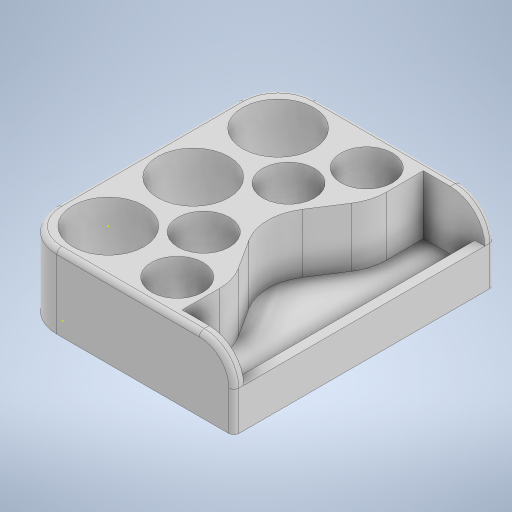
# Autodesk Inventor part: multi_battery_holder
Saved by Autodesk Inventor 2024 (Build 280153000, 153)
## iProperties
Created: 2024-03-18
Part Number: multi_battery_holder
Material: Generic
Document SubType Name: Modeling
Designer: kubad
Density: 1 g/cm^3
Appearance: Default
Author: kubad
Autodesk Inventor part; units mm, degrees
ref_plane "YZ Plane" through (0, 0, 0) normal (1, 0, 0) x (0, 1, 0)
ref_plane "XZ Plane" through (0, 0, 0) normal (0, 1, 0) x (-1, 0, 0)
ref_plane "XY Plane" through (0, 0, 0) normal (0, 0, 1) x (1, 0, 0)
sketch "Sketch1" plane through (0, 0, 0) normal (0, 1, 0) x (-1, 0, 0)
  circle A0 centre (0, 0) radius 7.25
  line L0 (0, -7.25) -> (0, -17.25)
  circle A1 centre (0, -17.25) radius 7.25
  line L1 (0, -24.5) -> (0, -34.5)
  circle A2 centre (0, -34.5) radius 7.25
  line L2 (0, -7.25) -> (0, -10)
  line L3 (0, -24.5) -> (0, -27.25)
  line L4 (0, 7.25) -> (-16, 7.25)
  line L5 (-16, 7.25) -> (-16, 2)
  circle A3 centre (-16, 2) radius 5.25
  line L6 (0, -41.75) -> (-16, -41.75)
  line L7 (-16, -41.75) -> (-16, -36.5)
  circle A4 centre (-16, -36.5) radius 5.25
  line L8 (0, -8.625) -> (-16, -8.625)
  line L9 (0, -25.875) -> (-16, -25.875)
  circle A5 centre (-10.75, -8.625) radius 5.25
  circle A6 centre (-10.75, -25.875) radius 5.25
  line L10 (-16, 7.25) -> (-22.25, 7.25)
  line L11 (-22.25, 7.25) -> (-32.75, 7.25)
  line L12 (-32.75, 7.25) -> (-32.75, -41.75)
  line L13 (-32.75, -41.75) -> (-22.25, -41.75)
  line L14 (-22.25, -41.75) -> (-22.25, 7.25)
  line L15 (7.25, 7.25) -> (9.25, 7.25)
  line L16 (9.25, 7.25) -> (9.25, 9.25)
  line L17 (-32.75, -41.75) -> (-32.75, -43.75)
  line L18 (-32.75, -43.75) -> (-34.75, -43.75)
  line L19 (9.25, 9.25) -> (-34.75, 9.25)
  line L20 (-34.75, 9.25) -> (-34.75, -43.75)
  line L21 (-34.75, -43.75) -> (9.25, -43.75)
  line L22 (9.25, -43.75) -> (9.25, 9.25)
  dimension "d0" = 14.5
  dimension "d14" = 10
  dimension "d15" = 14.5
  dimension "d16" = 10
  dimension "d17" = 14.5
  dimension "d23" = 16
  dimension "d24" = 5.25
  dimension "d25" = 10.5
  dimension "d26" = 16
  dimension "d27" = 5.25
  dimension "d28" = 10.5
  dimension "d29" = 10.5
  dimension "d31" = 6.25
  dimension "d32" = 10.5
  dimension "d33" = 2
  dimension "d34" = 2
  dimension "d35" = 2
  dimension "d36" = 2
  constraints: 46 end point, 8 horizontal, 6 centre point, 6 point on circle, 5 coincident, 5 vertical, 4 parallel, 4 perpendicular, 4 point on line, 2 midpoint, 1 tangent, 1 vertical alignment, 2 other
  measures "d0" diameter of A0
  measures "d14" distance of L0.start L0.end
  measures "d15" diameter of A1
  measures "d16" distance of L1.start L1.end
  measures "d17" diameter of A2
  measures "d23" distance of L4.start L4.end
  measures "d24" distance of L4.end L5.end
  measures "d25" diameter of A3
  measures "d26" distance of L6.start L6.end
  measures "d27" distance of L6.end L7.end
  measures "d28" diameter of A5
  measures "d29" diameter of A6
  measures "d31" distance of L4.end L10.end
  measures "d32" distance of L13.end L12.end
  measures "d33" distance of L15.start L15.end
  measures "d34" distance of L15.end L16.end
  measures "d35" distance of L12.end L17.end
  measures "d36" distance of L17.end L18.end
extrude "Extrusion1" add sketch "Sketch1" along normal blind 12
sketch "Sketch2" plane through (0, 0, 0) normal (0, -1, 0) x (1, 0, 0)
  line L0 (34.75, 9.25) -> (34.75, -43.75) projected
  line L1 (34.75, 9.25) -> (-9.25, 9.25)
  line L2 (-9.25, 9.25) -> (-9.25, -43.75)
  line L3 (-9.25, -43.75) -> (34.75, -43.75)
  line L4 (34.75, -43.75) -> (34.75, 9.25)
  point P0 (0, 0)
  constraints: 8 end point, 2 parallel, 1 horizontal, 1 perpendicular
extrude "Extrusion2" add sketch "Sketch2" along normal blind 3
sketch "Sketch3" plane through (0, 12, 0) normal (0, 1, 0) x (1, 0, 0)
  line L0 (32.75, 41.75) -> (32.75, -7.25) projected
  line L1 (32.75, 41.75) -> (34.75, 41.75)
  line L2 (34.75, -9.25) -> (34.75, 43.75) projected
  line L3 (32.75, -7.25) -> (34.75, -7.25)
  line L4 (34.75, -7.25) -> (34.75, 41.75)
  line L5 (34.75, 41.75) -> (32.75, 41.75)
  line L6 (32.75, 41.75) -> (32.75, -7.25)
  point P0 (0, 0)
  constraints: 10 end point, 2 horizontal, 2 parallel, 1 perpendicular, 1 point on line
extrude "Extrusion3" cut sketch "Sketch3" against normal blind 7
fillet "Fillet1" radius 7 1 edges at (34.75, 12, 8.25)
fillet "Fillet2" radius 7 1 edges at (34.75, 12, -42.75)
sketch "Sketch4" plane through (0, 12, 0) normal (0, 1, 0) x (1, 0, 0)
  line L0 (22.25, 41.75) -> (27.75, 41.75) projected
  line L1 (22.25, 41.75) -> (22.25, 31.25)
  line L2 (22.25, -7.25) -> (22.25, 41.75) projected
  line L3 (22.25, -7.25) -> (22.25, 3.25)
  line L4 (16, 17.25) -> (22.25, 31.25)
  line L5 (16, 17.25) -> (22.25, 3.25)
  line L6 (22.25, 17.25) -> (13.25, 17.25)
  line L7 (13.25, 17.25) -> (22.25, 31.25)
  line L8 (13.25, 17.25) -> (22.25, 3.25)
  line L9 (22.25, 31.25) -> (22.25, 3.25)
  point P0 (0, 0)
  dimension "d45" = 10.5
  dimension "d46" = 9
  constraints: 16 end point, 2 point on line, 1 collinear, 1 horizontal, 1 midpoint
  measures "d45" distance of L0.start L1.end
  measures "d46" distance of L6.start L6.end
extrude "Extrusion4" cut sketch "Sketch4" against normal blind 12 contours L6 L4 L2
extrude "Extrusion5" cut sketch "Sketch4" against normal blind 12 contours L5 L6 L2
extrude "Extrusion6" cut sketch "Sketch4" against normal blind 12 contours L8 L6 L5
extrude "Extrusion7" cut sketch "Sketch4" against normal through all contours L6 L7 L4
sketch "Sketch5" plane through (0, -3, 0) normal (0, -1, 0) x (1, 0, 0)
  line L0 (34.75, 9.25) -> (-9.25, 9.25)
  line L1 (-9.25, 9.25) -> (-9.25, -43.75)
  line L2 (-9.25, -43.75) -> (34.75, -43.75)
  line L3 (34.75, -43.75) -> (34.75, 9.25)
  point P0 (0, 0)
  constraints: 8 end point, 2 parallel, 1 horizontal, 1 perpendicular
extrude "Extrusion8" add sketch "Sketch5" against normal blind 3
fillet "Fillet3" radius 10 1 edges at (22.25, 6, -31.25)
fillet "Fillet4" radius 10 1 edges at (22.25, 6, -3.25)
fillet "Fillet5" radius 10 1 edges at (13.25, 6, -17.25)
sketch "Sketch6" plane through (-9.25, -3, 9.25) normal (0, 0, 1) x (1, 0, 0)
  point P0 (9.25, 3)
sketch "Sketch7" plane through (0, 12, 0) normal (0, 1, 0) x (1, 0, 0)
  point P0 (0, 0)
fillet "Fillet6" radius 8 1 edges at (-9.25, 4.5, 9.25)
fillet "Fillet7" radius 8 1 edges at (-9.25, 4.5, -43.75)
fillet "Fillet8" radius 1 9 edges at (32.6997, 9.9497, 9.25) (13.25, 12, 9.25) (-6.9069, 12, 6.9069) (-9.25, 12, -17.25) (-6.9069, 12, -41.4069) (13.25, 12, -43.75) (32.6997, 9.9497, -43.75) (34.75, 1, -43.75) (34.75, 1, 9.25)
body "Solid1"
